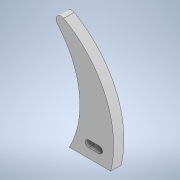
# Autodesk Inventor part: mavac_ruka I guesss
Saved by Autodesk Inventor 2022 (Build 260153000, 153)
## iProperties
Created: 2022-08-25
Part Number: mavac_ruka I guesss
Material: Generic
Document SubType Name: Modeling
Designer: Ruslana Zubareva
Density: 1 g/cm^3
Appearance: Default
Author: Ruslana Zubareva
Autodesk Inventor part; units mm, degrees
ref_plane "YZ Plane" through (0, 0, 0) normal (1, 0, 0) x (0, 1, 0)
ref_plane "XZ Plane" through (0, 0, 0) normal (0, 1, 0) x (-1, 0, 0)
ref_plane "XY Plane" through (0, 0, 0) normal (0, 0, 1) x (1, 0, 0)
sketch "Sketch1" plane through (0, 0, 0) normal (0, 0, 1) x (1, 0, 0)
  arc A0 (6.3455, 7.6592) -> (3.4138, 3.6532) centre (5.1207, 5.4798) ccw
  line L0 (18.4294, -37.0751) -> (23.4294, -37.0751)
  line L1 (23.4294, -40.2751) -> (18.4294, -40.2751)
  arc A1 (18.4294, -37.0751) -> (18.4294, -40.2751) centre (18.4294, -38.6751) ccw
  arc A2 (23.4294, -40.2751) -> (23.4294, -37.0751) centre (23.4294, -38.6751) ccw
  arc A3 (29.0127, -44.8588) -> (6.3455, 7.6592) centre (-16.7656, -33.4664) ccw
  arc A4 (9.0127, -44.8588) -> (3.4138, 3.6532) centre (-28.5567, -24.6156) ccw
  line L2 (9.0127, -44.8588) -> (29.0127, -44.8588)
  point P0 (0, 0)
  dimension "d20" = 3.2
  dimension "d25" = 2.5
  dimension "d32" = 20
  dimension "d35" = 5
  constraints: 10 point on circle, 6 end point, 5 centre point, 5 tangent, 2 parallel, 1 horizontal
  measures "d20" distance between parallel lines of L1 L0
  measures "d25" radius of A0
  measures "d32" distance of L2.start L2.end
  measures "d35" distance of A2.centre A1.centre
extrude "Extrusion1" add sketch "Sketch1" along normal blind 5
body "Solid1"
